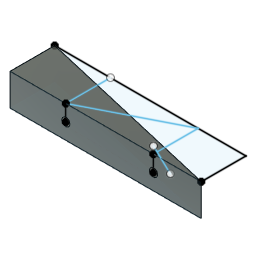
OsiguracZaPravUgao(TrougaoSaDveRupeM5) v2 (Autodesk Fusion 360 design; units mm, degrees)
Autodesk Fusion 360 part; units mm, degrees
note: some values were not read from the file. Set by a fixed rule: which sketch regions a step uses.
sketch "Sketch1" plane through (0, 0, 0) normal (0, 0, 1) x (1, 0, 0)
  line L0 (30, 50) -> (30, 22)
  line L1 (30, 22) -> (150, 22)
  line L2 (150, 22) -> (30, 50)
  dimension "d1" = 28
  dimension "d2" = 120
  constraint vertical L0
  constraint perpendicular L0 L1
  measures "d1" distance of L0.start L0.end
  measures "d2" distance of L0.end L1.end
extrude "Extrude1" add sketch "Sketch1" along normal blind 20
sketch "Sketch2" plane through (0, 22, 0) normal (0, -1, 0) x (1, 0, 0)
  line L0 (30, 0) -> (150, 0)
  line L1 (150, 0) -> (150, 20)
  line L2 (150, 20) -> (30, 20)
  line L3 (30, 20) -> (30, 0)
  line L4 (30, 10) -> (150, 10)
  line L5 (150, 10) -> (120, 10)
  circle A0 centre (120, 10) radius 2.5
  circle A1 centre (65, 10) radius 2.5
  dimension "d5" = 30
  dimension "d6" = 5
  dimension "d7" = 5
  constraint midpoint L3 L4.start
  constraint midpoint L1 L4.end
  constraint perpendicular L1 L5
  constraint coincident L5.end A0.centre
  constraint coincident L4 A1.centre
  measures "d5" distance of L4.end L5.end
  measures "d6" diameter of A0
  measures "d7" diameter of A1
extrude "Extrude2" cut sketch "Sketch2" against normal blind 50 contours L4 A1 | L4 A1 | L4 L5 A0 | L4 L5 A0
sketch "Sketch3" plane through (0, 0, 20) normal (0, 0, 1) x (-1, 0, 0)
  line L0 (-150, -22) -> (-30, -50)
  line L1 (-30, -50) -> (-30, -22)
  line L2 (-30, -22) -> (-150, -22)
  line L3 (-30, -50) -> (-150, -50)
  line L4 (-150, -50) -> (-150, -22)
  constraint coincident L0.end L1.start
  constraint perpendicular L1 L3
  constraint coincident L0.start L2.end
  constraint perpendicular L2 L4
sketch "Sketch4" plane through (0, 22, 0) normal (0, -1, 0) x (1, 0, 0)
  circle A0 centre (65, 10) radius 2.5
  circle A1 centre (120, 10) radius 2.5
  line L0 (30, 0) -> (150, 0)
  line L1 (150, 0) -> (150, 20)
  line L2 (150, 20) -> (30, 20)
  line L3 (30, 20) -> (30, 0)
  line L4 (65, 10) -> (65, 20)
  line L5 (120, 10) -> (120, 20)
  constraint coincident A0.centre L4.start
  constraint coincident L2 L4.end
  constraint perpendicular L2 L4
  constraint coincident A1.centre L5.start
  constraint coincident L2 L5.end
  constraint perpendicular L2 L5
sketch "Sketch5" plane through (0, 0, 20) normal (0, 0, 1) x (-1, 0, 0)
  line L0 (-120, -22) -> (-120, -50)
  line L1 (-120, -50) -> (-65, -22)
  line L2 (-65, -22) -> (-65, -50)
  constraint vertical L0
  constraint parallel L0 L2
sketch "Sketch6" plane through (90, 22, 10) normal (0, -1, 0) x (1, 0, 0)
  line L0 (30, 14.4) -> (40.6132, 4.6089)
sketch "Sketch7" plane through (0, 0, 0) normal (0, 0, -1) x (1, 0, 0)
  line L0 (30, -50) -> (150, -22)
  line L1 (150, -22) -> (30, -22)
  line L2 (30, -22) -> (30, -50)
